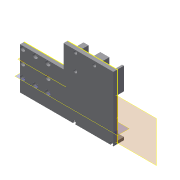
# Autodesk Inventor part: 10_MiniSPIM_Base_v1
Saved by Autodesk Inventor 2019 (Build 230136000, 136)
## iProperties
Created: 2019-10-10
Part Number: 10_MiniSPIM_Base_v1
Material: Generic
Document SubType Name: Modeling
Designer: diederichbenedict
Density: 1 g/cm^3
Appearance: Default
Author: diederichbenedict
Autodesk Inventor part; units mm, degrees
ref_plane "YZ Plane" through (0, 0, 0) normal (1, 0, 0) x (0, 1, 0)
ref_plane "XZ Plane" through (0, 0, 0) normal (0, 1, 0) x (-1, 0, 0)
ref_plane "XY Plane" through (0, 0, 0) normal (0, 0, 1) x (1, 0, 0)
ref_plane "Work Plane1" through (0, 0, 3) normal (0, 0, 1) x (1, 0, 0)
sketch "Sketch1" plane through (0, 0, 3) normal (0, 0, 1) x (1, 0, 0)
  line L0 (73, -36.65) -> (-73, -36.65) construction
  line L1 (73, 36.65) -> (73, -36.65) construction
  line L2 (-73, 36.65) -> (73, 36.65) construction
  line L3 (-73, -36.65) -> (-73, 36.65) construction
  line L4 (-66.8632, 12.8749) -> (-66.8632, 14.232) construction
  line L5 (-66.8632, 14.232) -> (-61.4969, 10.9795) construction
  line L6 (-61.4969, 10.9795) -> (-57.2382, 10.9795) construction
  line L7 (-57.2382, 10.9795) -> (-57.2382, 9.7003) construction
  line L8 (-57.2382, 9.7003) -> (-61.3643, 9.7003) construction
  line L9 (-61.3643, 9.7003) -> (-66.8632, 6.4478) construction
  line L10 (-66.8632, 6.4478) -> (-66.8632, 7.8674) construction
  line L11 (-66.8632, 7.8674) -> (-62.6279, 10.3477) construction
  line L12 (-62.6279, 10.3477) -> (-66.8632, 12.8749) construction
  spline S0 degree 2 poles (-57.9402, -12.888) (-57.519, -13.3482) (-57.0666, -14.5182) (-57.0666, -15.3995) knots 0 0 0 1 2 2 2 construction
  spline S1 degree 2 poles (-57.0666, -15.3995) (-57.0666, -16.4447) (-57.5034, -17.9111) (-57.8154, -18.5585) knots 0 0 0 1 2 2 2 construction
  line L13 (-57.8154, -18.5585) -> (-59.4221, -18.5585) construction
  line L14 (-59.4221, -18.5585) -> (-59.4221, -18.4649) construction
  spline S2 degree 2 poles (-59.4221, -18.4649) (-58.8294, -17.8331) (-58.1742, -16.2341) (-58.1742, -15.4931) knots 0 0 0 1 2 2 2 construction
  spline S3 degree 2 poles (-58.1742, -15.4931) (-58.1742, -14.4324) (-59.0555, -13.3482) (-59.7809, -13.3482) knots 0 0 0 1 2 2 2 construction
  spline S4 degree 2 poles (-59.7809, -13.3482) (-60.3581, -13.3482) (-61.0757, -13.9176) (-61.2551, -14.5338) knots 0 0 0 1 2 2 2 construction
  spline S5 degree 2 poles (-61.2551, -14.5338) (-61.3799, -14.9784) (-61.5515, -15.7193) (-61.6919, -16.2731) knots 0 0 0 1 2 2 2 construction
  spline S6 degree 2 poles (-61.6919, -16.2731) (-61.8245, -16.7723) (-62.2223, -17.5601) (-62.5421, -17.8643) knots 0 0 0 1 2 2 2 construction
  spline S7 degree 2 poles (-62.5421, -17.8643) (-62.8619, -18.1607) (-63.7199, -18.4883) (-64.2814, -18.4883) knots 0 0 0 1 2 2 2 construction
  spline S8 degree 2 poles (-64.2814, -18.4883) (-65.4514, -18.4883) (-67.0348, -16.6631) (-67.0348, -15.2514) knots 0 0 0 1 2 2 2 construction
  spline S9 degree 2 poles (-67.0348, -15.2514) (-67.0348, -14.4402) (-66.715, -13.005) (-66.4108, -12.3888) knots 0 0 0 1 2 2 2 construction
  line L15 (-66.4108, -12.3888) -> (-64.882, -12.3888) construction
  line L16 (-64.882, -12.3888) -> (-64.882, -12.4824) construction
  spline S10 degree 2 poles (-64.882, -12.4824) (-65.3032, -12.9426) (-65.9272, -14.3778) (-65.9272, -15.1656) knots 0 0 0 1 2 2 2 construction
  spline S11 degree 2 poles (-65.9272, -15.1656) (-65.9272, -16.0547) (-65.0926, -17.1545) (-64.414, -17.1545) knots 0 0 0 1 2 2 2 construction
  spline S12 degree 2 poles (-64.414, -17.1545) (-63.8057, -17.1545) (-63.0803, -16.5071) (-62.9165, -15.8987) knots 0 0 0 1 2 2 2 construction
  spline S13 degree 2 poles (-62.9165, -15.8987) (-62.8073, -15.4931) (-62.5265, -14.3154) (-62.4095, -13.9254) knots 0 0 0 1 2 2 2 construction
  spline S14 degree 2 poles (-62.4095, -13.9254) (-62.1053, -12.9348) (-60.8807, -12.0144) (-59.9837, -12.0144) knots 0 0 0 1 2 2 2 construction
  spline S15 degree 2 poles (-59.9837, -12.0144) (-59.4143, -12.0144) (-58.3224, -12.4746) (-57.9402, -12.888) knots 0 0 0 1 2 2 2 construction
  spline S16 degree 2 poles (-67.066, -7.0069) (-67.066, -6.0241) (-66.3796, -4.4486) (-65.7634, -3.9026) knots 0 0 0 1 2 2 2 construction
  spline S17 degree 2 poles (-65.7634, -3.9026) (-65.1238, -3.3566) (-63.2519, -2.7482) (-62.0507, -2.7482) knots 0 0 0 1 2 2 2 construction
  spline S18 degree 2 poles (-62.0507, -2.7482) (-60.8807, -2.7482) (-58.9854, -3.341) (-58.3458, -3.9026) knots 0 0 0 1 2 2 2 construction
  spline S19 degree 2 poles (-58.3458, -3.9026) (-57.675, -4.4954) (-57.0354, -6.0631) (-57.0354, -7.0069) knots 0 0 0 1 2 2 2 construction
  spline S20 degree 2 poles (-57.0354, -7.0069) (-57.0354, -7.9819) (-57.6984, -9.5419) (-58.3458, -10.1113) knots 0 0 0 1 2 2 2 construction
  spline S21 degree 2 poles (-58.3458, -10.1113) (-58.9854, -10.665) (-60.8651, -11.2578) (-62.0507, -11.2578) knots 0 0 0 1 2 2 2 construction
  spline S22 degree 2 poles (-62.0507, -11.2578) (-63.2597, -11.2578) (-65.1004, -10.6572) (-65.7634, -10.1035) knots 0 0 0 1 2 2 2 construction
  spline S23 degree 2 poles (-65.7634, -10.1035) (-66.403, -9.5419) (-67.066, -7.9741) (-67.066, -7.0069) knots 0 0 0 1 2 2 2 construction
  line L17 (-66.8632, 5.543) -> (-57.2382, 5.543) construction
  line L18 (-57.2382, 5.543) -> (-57.2382, 4.1078) construction
  line L19 (-57.2382, 4.1078) -> (-65.5372, -0.1509) construction
  line L20 (-65.5372, -0.1509) -> (-57.2382, -0.1509) construction
  line L21 (-57.2382, -0.1509) -> (-57.2382, -1.3442) construction
  line L22 (-57.2382, -1.3442) -> (-66.8632, -1.3442) construction
  line L23 (-66.8632, -1.3442) -> (-66.8632, 0.4731) construction
  line L24 (-66.8632, 0.4731) -> (-59.2427, 4.3496) construction
  line L25 (-59.2427, 4.3496) -> (-66.8632, 4.3496) construction
  line L26 (-66.8632, 4.3496) -> (-66.8632, 5.543) construction
  circle A0 centre (-154.415, -17.3382) radius 1.95 construction
  circle A1 centre (-129.415, 7.6618) radius 1.95 construction
  circle A2 centre (-129.415, 32.6618) radius 1.95 construction
  circle A3 centre (-179.415, -17.3382) radius 1.95 construction
  circle A4 centre (-179.415, 32.6618) radius 1.95 construction
  circle A5 centre (-129.415, -17.3382) radius 1.95 construction
  circle A6 centre (-179.415, 7.6618) radius 1.95 construction
  circle A7 centre (-154.415, 32.6618) radius 1.95 construction
  line L27 (-126.415, -22.3382) -> (-124.415, -20.3382) construction
  line L28 (-124.415, -20.3382) -> (-124.415, 35.6618) construction
  line L29 (-124.415, 35.6618) -> (-126.415, 37.6618) construction
  line L30 (-126.415, 37.6618) -> (-182.415, 37.6618) construction
  line L31 (-182.415, 37.6618) -> (-184.415, 35.6618) construction
  line L32 (-184.415, 35.6618) -> (-184.415, -20.3382) construction
  line L33 (-184.415, -20.3382) -> (-182.415, -22.3382) construction
  line L34 (-182.415, -22.3382) -> (-126.415, -22.3382) construction
  circle A8 centre (-93.2, 28.85) radius 2.1512 construction
  arc A9 (-95.5, 82.55) -> (-98.5, 79.55) centre (-95.5, 79.55) ccw construction
  line L35 (-98.5, 18.65) -> (-98.5, 79.55) construction
  arc A10 (-98.5, 18.65) -> (-95.5, 15.65) centre (-95.5, 18.65) ccw construction
  line L36 (39.6, 15.65) -> (-95.5, 15.65) construction
  arc A11 (39.6, 15.65) -> (42.6, 18.65) centre (39.6, 18.65) ccw construction
  line L37 (42.6, 79.55) -> (42.6, 18.65) construction
  arc A12 (42.6, 79.55) -> (39.6, 82.55) centre (39.6, 79.55) ccw construction
  line L38 (-95.5, 82.55) -> (39.6, 82.55) construction
  line L39 (-184.415, -44.9655) -> (0, -44.9655)
  line L40 (0, -44.9655) -> (0, 82.55)
  line L41 (0, 82.55) -> (-184.415, 82.55)
  line L42 (-184.415, 82.55) -> (-184.415, -44.9655)
  circle A13 centre (-179.415, 32.6618) radius 2.95
  circle A14 centre (-154.415, 32.6618) radius 2.95
  circle A15 centre (-129.415, 32.6618) radius 2.95
  circle A16 centre (-129.415, 7.6618) radius 2.95
  circle A17 centre (-129.415, -17.3382) radius 2.95
  circle A18 centre (-154.415, -17.3382) radius 2.95
  circle A19 centre (-179.415, -17.3382) radius 2.95
  circle A20 centre (-179.415, 7.6618) radius 2.95
  line L43 (-184.415, 82.55) -> (-98.5, 82.55)
  line L44 (-98.5, 82.55) -> (-98.5, 37.6618)
  line L45 (-98.5, 37.6618) -> (-184.415, 37.6618)
  line L46 (-184.415, 37.6618) -> (-184.415, 82.55)
  point P0 (0, 0)
  dimension "d0" = 1
  dimension "d1" = 1
  dimension "d2" = 1
  dimension "d3" = 1
  dimension "d4" = 1
  dimension "d5" = 1
  dimension "d6" = 1
  dimension "d7" = 1
  constraints: 16 end point, 8 centre point, 4 parallel, 2 horizontal, 2 perpendicular, 2 point on line
  measures "d0" radial gap between concentric circles of A4 A13
  measures "d1" radial gap between concentric circles of A7 A14
  measures "d2" radial gap between concentric circles of A2 A15
  measures "d3" radial gap between concentric circles of A1 A16
  measures "d4" radial gap between concentric circles of A5 A17
  measures "d5" radial gap between concentric circles of A0 A18
  measures "d6" radial gap between concentric circles of A3 A19
  measures "d7" radial gap between concentric circles of A6 A20
ref_plane "Work Plane2" through (-73, -36.65, 0) normal (0, 0, 1) x (1, 0, 0)
extrude "Extrusion1" add sketch "Sketch1" along normal blind 5 and the other way blind 3 contours L42 L45 L44 L41 L40 L39
sketch "Sketch2" plane through (0, 0, 0) normal (0, 0, -1) x (1, 0, 0)
  line L0 (-184.415, -37.6618) -> (-98.5, -37.6618) projected
  line L1 (-184.415, 44.9655) -> (-184.415, -37.6618) projected
  line L2 (0, 44.9655) -> (-184.415, 44.9655) projected
  line L3 (0, -82.55) -> (0, 44.9655) projected
  line L4 (-98.5, -82.55) -> (0, -82.55) projected
  line L5 (-98.5, -37.6618) -> (-98.5, -82.55) projected
  circle A0 centre (-179.415, -7.6618) radius 2.95 projected
  circle A1 centre (-179.415, 17.3382) radius 2.95 projected
  circle A2 centre (-154.415, 17.3382) radius 2.95 projected
  circle A3 centre (-129.415, 17.3382) radius 2.95 projected
  circle A4 centre (-129.415, -7.6618) radius 2.95 projected
  circle A5 centre (-129.415, -32.6618) radius 2.95 projected
  circle A6 centre (-154.415, -32.6618) radius 2.95 projected
  circle A7 centre (-179.415, -32.6618) radius 2.95 projected
  point P0 (0, 0)
sketch "Sketch3" plane through (0, 0, 8) normal (0, 0, 1) x (1, 0, 0)
  line L0 (-98.5, 82.55) -> (-98.5, 37.6618) projected
  line L1 (-98.5, 37.6618) -> (-184.415, 37.6618) projected
  line L2 (-184.415, 37.6618) -> (-184.415, -44.9655) projected
  line L3 (-184.415, -44.9655) -> (0, -44.9655) projected
  line L4 (0, -44.9655) -> (0, 82.55) projected
  line L5 (0, 82.55) -> (-98.5, 82.55) projected
  circle A0 centre (-179.415, 32.6618) radius 2.95 projected
  circle A1 centre (-154.415, 32.6618) radius 2.95 projected
  circle A2 centre (-129.415, 32.6618) radius 2.95 projected
  circle A3 centre (-129.415, 7.6618) radius 2.95 projected
  circle A4 centre (-129.415, -17.3382) radius 2.95 projected
  circle A5 centre (-154.415, -17.3382) radius 2.95 projected
  circle A6 centre (-179.415, -17.3382) radius 2.95 projected
  circle A7 centre (-179.415, 7.6618) radius 2.95 projected
  point P0 (0, 0)
hole "Hole1" at (-179.415, 32.6618, 8) at (-154.415, 32.6618, 8) at (-129.415, 32.6618, 8) at (-129.415, 7.6618, 8) at (-129.415, -17.3382, 8) at (-154.415, -17.3382, 8) at (-179.415, -17.3382, 8) at (-179.415, 7.6618, 8) direction (0, 0, -1) diameter 5.3 depth 10 tip angle 118 counterbore diameter 10 counterbore depth 5
sketch "Sketch4" plane through (0, 0, 0) normal (0, 0, -1) x (-1, 0, 0)
  line L0 (-75, -38.65) -> (75, -38.65) projected
  line L1 (75, 38.65) -> (-75, 38.65) projected
  line L2 (0, -44.9655) -> (184.415, -44.9655) projected
  line L3 (0, -44.9655) -> (75, -44.9655)
  line L4 (75, -44.9655) -> (75, -39.3793)
  line L5 (75, -39.3793) -> (0, -39.3793)
  line L6 (0, -39.3793) -> (0, -44.9655)
  line L7 (98.5, 82.55) -> (0, 82.55) projected
  line L8 (0, 82.55) -> (3.6448, 82.55)
  line L9 (3.6448, 82.55) -> (3.6448, 38.65)
  line L10 (3.6448, 38.65) -> (0, 38.65)
  line L11 (0, 38.65) -> (0, 82.55)
  line L12 (33.963, 38.65) -> (28.963, 38.65)
  line L13 (28.963, 38.65) -> (28.963, 82.55)
  line L14 (28.963, 82.55) -> (33.963, 82.55)
  line L15 (33.963, 82.55) -> (33.963, 38.65)
  line L16 (70, 38.65) -> (75, 38.65)
  line L17 (75, 38.65) -> (75, 82.55)
  line L18 (75, 82.55) -> (70, 82.55)
  line L19 (70, 82.55) -> (70, 38.65)
  line L20 (75, -44.9655) -> (80, -44.9655)
  line L21 (80, -44.9655) -> (80, -8.9655)
  line L22 (80, -8.9655) -> (75, -8.9655)
  line L23 (75, -8.9655) -> (75, -44.9655)
  line L24 (75, 82.55) -> (80, 82.55)
  line L25 (80, 82.55) -> (80, 32.55)
  line L26 (80, 32.55) -> (75, 32.55)
  line L27 (75, 32.55) -> (75, 82.55)
  line L28 (0, 38.65) -> (75, 38.65)
  line L29 (75, 38.65) -> (75, 39.65)
  line L30 (75, 39.65) -> (0, 39.65)
  line L31 (0, 39.65) -> (0, 38.65)
  line L32 (75, -8.9655) -> (107, -8.9655)
  line L33 (107, -8.9655) -> (107, -3.9655)
  line L34 (107, -3.9655) -> (75, -3.9655)
  line L35 (75, -3.9655) -> (75, -8.9655)
  line L36 (33.963, 82.55) -> (46.7902, 82.55)
  line L37 (46.7902, 82.55) -> (46.7902, 67.4779)
  line L38 (46.7902, 67.4779) -> (33.963, 67.4779)
  line L39 (33.963, 67.4779) -> (33.963, 82.55)
  point P0 (0, 0)
  point P1 (70, 39.65)
  point P2 (33.963, 39.65)
  point P3 (28.963, 39.65)
  point P4 (3.6448, 39.65)
  dimension "d19" = 5
  dimension "d20" = 36
  dimension "d21" = 50
  dimension "d22" = 5
  dimension "d23" = 5
  dimension "d24" = 1
  dimension "d41" = 32
  dimension "d42" = 5
  constraints: 72 end point, 18 parallel, 16 point on line, 9 horizontal, 9 perpendicular, 1 coincident
  measures "d19" distance of L22.end L21.end
  measures "d20" distance of L21.end L20.end
  measures "d21" distance of L24.end L25.end
  measures "d22" distance between parallel lines of L13 L15
  measures "d23" distance between parallel lines of L19 L17
  measures "d24" distance of L29.end L28.end
  measures "d41" distance of L34.end L33.end
  measures "d42" distance of L33.end L32.end
ref_plane "Work Plane3" through (-73, -36.65, -13.1) normal (0, 0, -1) x (0, 1, 0)
extrude "Extrusion2" add sketch "Sketch4" along normal up to surface (13.1 mm away) contours L1 L19 L30 L17 | L17 L7 L25 L26 L27 | L1 L15 L30 L19 | L30 L19 L7 L17 | L1 L13 L30 L15 | L1 L9 L30 L13 | L30 L13 L7 L15 | L1 L11 L30 L9 | L15 L7 L37 L38 | L30 L11 L7 L9 | L6 L5 L4 L2 | L4 L23 L22 L21 L2 | L22 L35 L34 L33 L32
ref_plane "Work Plane4" through (-184.415, -21.1655, 8) normal (0, -1, 0) x (1, 0, 0)
sketch "Sketch5" plane through (-184.415, -21.1655, 8) normal (0, -1, 0) x (1, 0, 0)
  line L0 (106.215, -7.26) -> (106.215, -19.94) projected
  arc A0 (109.315, -13.6) -> (107.415, -7.26) centre (94.5273, -14.5769) ccw
  arc A1 (107.415, -19.94) -> (109.315, -13.6) centre (94.5273, -12.6231) ccw
  line L1 (107.415, -7.26) -> (106.215, -7.26)
  line L2 (107.415, -19.94) -> (106.215, -19.94)
  arc A2 (109.6156, -13.6) -> (107.5884, -6.96) centre (94.5273, -14.5769) ccw
  line L3 (107.5884, -6.96) -> (105.915, -6.96)
  line L4 (105.915, -6.96) -> (105.915, -20.24)
  line L5 (105.915, -20.24) -> (107.5884, -20.24)
  arc A3 (107.5884, -20.24) -> (109.6156, -13.6) centre (94.5273, -12.6231) ccw
  line L6 (105.915, -19.2866) -> (104.415, -19.2866)
  line L7 (104.415, -8) -> (104.415, -21.1) projected
  line L8 (104.415, -13.6) -> (105.915, -13.6)
  line L9 (108.0996, -19.2866) -> (109.415, -19.2866)
  line L10 (109.415, -8) -> (109.415, -21.1) projected
  line L11 (105.915, -13.6) -> (109.6156, -13.6)
  line L12 (104.415, -8) -> (105.915, -8)
  line L13 (108.1418, -8) -> (109.415, -8)
  line L14 (109.415, -8) -> (109.415, -11.9371)
  line L15 (109.415, -11.9371) -> (109.415, -13.6)
  arc A4 (105.915, -6.96) -> (105.915, -20.24) centre (128.582, -13.6) ccw
  line L16 (104.9624, -13.6) -> (105.915, -13.6)
  line L17 (106.215, -7.26) -> (105.915, -7.26)
  line L18 (106.215, -19.94) -> (105.915, -19.94)
  point P0 (184.415, -8)
  dimension "d28" = 0.3
  constraints: 32 end point, 14 point on circle, 11 point on line, 5 centre point, 4 horizontal, 2 collinear, 2 parallel, 2 perpendicular, 1 coincident, 1 midpoint, 11 other
  measures "d28" radial gap between concentric circles of A1 A3
revolve "Revolution1" cut sketch "Sketch5" angle 360 about axis through (-80, -21.1655, -5.6) along (1, 0, 0) contours L1 A0 L11 L0 | L17 L4 L3 A2 L10 L11 A0 L1 | L0 L11 L4 L17 | L8 A4 L12 L4 | L8 L7 L12 A4 | L10 A2 L11 | A2 L13 L10
sketch "Sketch6" plane through (0, -44.9655, -13.1) normal (0, 0, -1) x (-1, 0, 0)
  line L0 (78.5, 17.16) -> (78.5, 30.44) projected
  line L1 (76.8265, 17.16) -> (78.5, 17.16) projected
  line L2 (76.8265, 30.44) -> (78.5, 30.44) projected
  arc A0 (77, 30.1555) -> (75.1, 23.8155) centre (89.8876, 22.8386) ccw
  arc A1 (75.1, 23.8155) -> (77, 17.4755) centre (89.8876, 24.7925) ccw
  line L3 (76.2622, 30.8555) -> (79.2, 30.8555)
  line L4 (79.2, 30.8555) -> (79.2, 16.46)
  line L5 (79.2, 16.46) -> (76.2622, 16.46)
  line L6 (76.2622, 16.46) -> (76.2622, 30.8555)
  line L7 (76.2622, 30.8555) -> (79.2, 16.46) construction
  line L8 (79.2, 30.8555) -> (76.2622, 16.46) construction
  arc A2 (76.2622, 30.8555) -> (76.2622, 16.46) centre (91.2579, 23.6578) ccw
  arc A3 (78.5, 16.46) -> (78.5, 30.8555) centre (55.9892, 23.6578) ccw
  point P0 (0, 44.9655)
  point P1 (77.7311, 23.6578)
  dimension "d30" = 0.7
  dimension "d31" = 0.7
  dimension "d32" = 0.7
  constraints: 12 end point, 8 point on circle, 4 centre point, 2 midpoint, 2 parallel, 2 point on line, 1 horizontal, 1 perpendicular, 7 other
  measures "d30" distance between parallel lines of L1 L5
  measures "d31" distance from line of L3 A0.start
  measures "d32" distance between parallel lines of L4 L0
extrude "Extrusion3" cut sketch "Sketch6" against normal blind 7
ref_plane "Work Plane5" through (-184.415, 10.1618, 0) normal (0, 1, 0) x (1, 0, 0)
sketch "Sketch8" plane through (0, 0, 0) normal (0, 0, -1) x (-1, 0, 0)
  point P0 (0, 0)
ref_plane "Work Plane6" through (-92.97, -44.9655, -13.1) normal (-1, 0, 0) x (0, 0, 1)
sketch "Sketch9" plane through (-92.97, -44.9655, -13.1) normal (-1, 0, 0) x (0, 0, 1)
  line L0 (1.5, 45.9155) -> (1.5, 30.5155) construction
  line L1 (-1.25, 45.9155) -> (16.25, 45.9155) construction
  line L2 (-1.25, 50.6155) -> (-1.25, 45.9155) construction
  arc A0 (7, 53.5251) -> (-1.25, 50.6155) centre (7, 40.3737) ccw construction
  line L3 (1.5, 30.5155) -> (13.5, 30.5155) construction
  line L4 (13.5, 45.9155) -> (13.5, 30.5155) construction
  arc A1 (16.25, 50.6155) -> (8, 53.5251) centre (8, 40.3737) ccw construction
  line L5 (13.1, 41) -> (0, 41) projected
  line L6 (7.5, 23.7837) -> (1.5, 23.7837)
  line L7 (1.5, 23.7837) -> (1.5, 41)
  line L8 (1.5, 41) -> (7.5, 41)
  line L9 (7.5, 41) -> (7.5, 23.7837)
  line L10 (7.5, 41) -> (-4.503, 41)
  line L11 (-4.503, 41) -> (-4.503, 60.9686)
  line L12 (-4.503, 60.9686) -> (7.5, 60.9686)
  line L13 (7.5, 60.9686) -> (7.5, 41)
  point P0 (13.1, 44.9655)
  constraints: 22 end point, 4 parallel, 4 point on circle, 3 vertical, 2 centre point, 2 horizontal, 2 perpendicular, 2 point on line, 11 other
revolve "Revolution2" cut sketch "Sketch9" angle 360 about axis through (-92.97, -3.9655, -5.6) along (0, -1, 0)
sketch "Sketch10" plane through (-80, 32.55, 0) normal (-1, 0, 0) x (0, 0, 1)
  line L0 (-1.3574, -6.5284) -> (-8.4284, 0.5426) projected
  line L1 (0, -77.5155) -> (0, 5.1118) projected
  line L2 (0, -7.8858) -> (-12.9976, 5.1118)
  line L3 (-12.9976, 5.1118) -> (0, 5.1118)
  line L4 (0, 5.1118) -> (0, -7.8858)
  point P0 (0, -32.55)
  constraints: 6 end point, 1 collinear, 1 perpendicular, 1 point on line
extrude "Extrusion5" add sketch "Sketch10" along normal up to surface (18.5 mm away)
sketch "Sketch11" plane through (0, 0, 8) normal (0, 0, 1) x (1, 0, 0)
  circle A0 centre (-154.415, -17.3382) radius 5 projected
  circle A1 centre (-129.415, 7.6618) radius 5 projected
  circle A2 centre (-129.415, -17.3382) radius 5 projected
  arc A3 (-184.415, 32.6618) -> (-179.415, 37.6618) centre (-179.415, 32.6618) ccw projected
  line L0 (-184.415, 32.6618) -> (-184.415, 7.6618) projected
  circle A4 centre (-179.415, 7.6618) radius 5 projected
  line L1 (-184.415, 7.6618) -> (-184.415, -17.3382) projected
  circle A5 centre (-179.415, -17.3382) radius 5 projected
  line L2 (-184.415, -17.3382) -> (-184.415, -44.9655) projected
  line L3 (-184.415, -44.9655) -> (0, -44.9655) projected
  line L4 (0, -44.9655) -> (0, 82.55) projected
  line L5 (0, 82.55) -> (-98.5, 82.55) projected
  line L6 (-98.5, 82.55) -> (-98.5, 37.6618) projected
  line L7 (-98.5, 37.6618) -> (-129.415, 37.6618) projected
  circle A6 centre (-129.415, 32.6618) radius 5 projected
  line L8 (-129.415, 37.6618) -> (-154.415, 37.6618) projected
  circle A7 centre (-154.415, 32.6618) radius 5 projected
  line L9 (-154.415, 37.6618) -> (-179.415, 37.6618) projected
  line L10 (-28.963, 82.55) -> (-46.7902, 82.55) projected
  line L11 (-28.963, 39.65) -> (-28.963, 82.55) projected
  line L12 (-3.6448, 39.65) -> (-28.963, 39.65) projected
  line L13 (-3.6448, 82.55) -> (-3.6448, 39.65) projected
  line L14 (0, 82.55) -> (-3.6448, 82.55) projected
  line L15 (0, 38.65) -> (0, 82.55) projected
  line L16 (-75, 38.65) -> (0, 38.65) projected
  line L17 (-75, 32.55) -> (-75, 38.65) projected
  line L18 (-80, 32.55) -> (-75, 32.55) projected
  line L19 (-80, 82.55) -> (-80, 32.55) projected
  line L20 (-70, 82.55) -> (-80, 82.55) projected
  line L21 (-70, 39.65) -> (-70, 82.55) projected
  line L22 (-33.963, 39.65) -> (-70, 39.65) projected
  line L23 (-33.963, 67.4779) -> (-33.963, 39.65) projected
  arc A8 (-75, -17.7921) -> (-76.2622, -14.11) centre (-91.2579, -21.3078) ccw projected
  line L24 (-76.2622, -14.11) -> (-79.2, -14.11) projected
  line L25 (-79.2, -14.11) -> (-79.2, -16.8577) projected
  arc A9 (-79.2, -16.8577) -> (-79.2, -25.7578) centre (-55.9892, -21.3078) ccw projected
  line L26 (-79.2, -25.7578) -> (-79.2, -28.5055) projected
  line L27 (-79.2, -28.5055) -> (-76.2622, -28.5055) projected
  arc A10 (-76.2622, -28.5055) -> (-75, -24.8235) centre (-91.2579, -21.3078) ccw projected
  line L28 (-75, -39.3793) -> (-75, -24.8235) projected
  line L29 (0, -39.3793) -> (-75, -39.3793) projected
  line L30 (0, -44.9655) -> (0, -39.3793) projected
  line L31 (-80, -44.9655) -> (0, -44.9655) projected
  line L32 (-80, -8.9655) -> (-80, -44.9655) projected
  line L33 (-107, -8.9655) -> (-80, -8.9655) projected
  line L34 (-107, -3.9655) -> (-107, -8.9655) projected
  line L35 (-75, -3.9655) -> (-107, -3.9655) projected
  line L36 (-75, -17.7921) -> (-75, -3.9655) projected
  line L37 (-46.7902, 67.4779) -> (-33.963, 67.4779) projected
  line L38 (-46.7902, 82.55) -> (-46.7902, 67.4779) projected
  point P0 (0, 0)
  point P1 (-75, 78.2799)
  point P2 (-75, 46.097)
  point P3 (-77.7311, -42.1724)
  point P4 (-3.6448, -42.1724)
  point P5 (-37.5, 75.014)
  constraints: 2 horizontal alignment, 2 vertical alignment
hole "Hole2" at (-75, 78.2799, 8) at (-75, 46.097, 8) at (-77.7311, -42.1724, 8) at (-3.6448, -42.1724, 8) at (-37.5, 75.014, 8) direction (0, 0, -1) diameter 3.3 end through all counterbore diameter 6.8 counterbore depth 5
sketch "Sketch12" plane through (0, 0, 0) normal (0, 0, -1) x (-1, 0, 0)
  line L0 (80, 24.6642) -> (80, 32.55) projected
  line L1 (80, 32.55) -> (75, 32.55) projected
  line L2 (75, 32.55) -> (75, 38.65) projected
  line L3 (75, 38.65) -> (0, 38.65) projected
  line L4 (0, 38.65) -> (0, -39.3793) projected
  line L5 (0, -39.3793) -> (75, -39.3793) projected
  line L6 (75, -39.3793) -> (75, -21.1655) projected
  line L7 (75, -21.1655) -> (75, -3.9655) projected
  line L8 (75, -3.9655) -> (82.3534, -3.9655) projected
  line L9 (82.3534, -3.9655) -> (82.3534, 16.003) projected
  line L10 (82.3534, 16.003) -> (103.5866, 16.003) projected
  line L11 (103.5866, 16.003) -> (103.5866, -3.9655) projected
  line L12 (103.5866, -3.9655) -> (107, -3.9655) projected
  line L13 (107, -3.9655) -> (107, -8.9655) projected
  line L14 (107, -8.9655) -> (95.1241, -8.9655) projected
  line L15 (95.1241, -8.9655) -> (95.1241, -21.1818) projected
  line L16 (95.1241, -21.1818) -> (90.8159, -21.1818) projected
  line L17 (90.8159, -21.1818) -> (90.8159, -8.9655) projected
  line L18 (90.8159, -8.9655) -> (80, -8.9655) projected
  line L19 (80, -8.9655) -> (80, -21.1655) projected
  line L20 (80, -21.1655) -> (80, -44.9655) projected
  line L21 (80, -44.9655) -> (184.415, -44.9655) projected
  line L22 (184.415, -44.9655) -> (184.415, 37.6618) projected
  line L23 (184.415, 37.6618) -> (98.5, 37.6618) projected
  line L24 (98.5, 37.6618) -> (98.5, 24.6642) projected
  line L25 (98.5, 24.6642) -> (80, 24.6642) projected
  circle A0 centre (179.415, 7.6618) radius 2.95 projected
  circle A1 centre (179.415, -17.3382) radius 2.95 projected
  circle A2 centre (154.415, -17.3382) radius 2.95 projected
  circle A3 centre (129.415, -17.3382) radius 2.95 projected
  circle A4 centre (129.415, 7.6618) radius 2.95 projected
  circle A5 centre (129.415, 32.6618) radius 2.95 projected
  circle A6 centre (154.415, 32.6618) radius 2.95 projected
  circle A7 centre (179.415, 32.6618) radius 2.95 projected
  line L26 (126.415, -22.3382) -> (124.415, -20.3382) projected
  line L27 (126.415, -22.3382) -> (182.415, -22.3382) projected
  line L28 (184.415, -20.3382) -> (182.415, -22.3382) projected
  line L29 (184.415, -20.3382) -> (184.415, 35.6618) projected
  line L30 (182.415, 37.6618) -> (184.415, 35.6618) projected
  line L31 (182.415, 37.6618) -> (126.415, 37.6618) projected
  line L32 (124.415, 35.6618) -> (126.415, 37.6618) projected
  line L33 (124.415, 35.6618) -> (124.415, -20.3382) projected
  circle A8 centre (129.415, 7.6618) radius 1.3 projected
  circle A9 centre (179.415, 7.6618) radius 1.3 projected
  circle A10 centre (154.415, 7.6618) radius 7.5 projected
  line L34 (107, -8.9655) -> (80, -8.9655) projected
  line L35 (184.415, -44.9655) -> (79.6698, -44.9655) projected
  line L36 (80, -8.9655) -> (124.415, -8.9655)
  line L37 (124.415, -8.9655) -> (124.415, -44.9655)
  line L38 (124.415, -44.9655) -> (80, -44.9655)
  line L39 (80, -44.9655) -> (80, -8.9655)
  line L40 (184.415, -44.9655) -> (124.415, -44.9655)
  line L41 (124.415, -44.9655) -> (124.415, -22.3382)
  line L42 (124.415, -22.3382) -> (184.415, -22.3382)
  line L43 (184.415, -22.3382) -> (184.415, -44.9655)
  line L44 (90.8159, -21.1818) -> (95.1241, -21.1818)
  line L45 (95.1241, -21.1818) -> (95.1241, -8.9655)
  line L46 (95.1241, -8.9655) -> (90.8159, -8.9655)
  line L47 (90.8159, -8.9655) -> (90.8159, -21.1818)
  point P0 (0, 0)
  constraints: 24 end point, 6 parallel, 3 horizontal, 3 perpendicular, 2 point on line
extrude "Extrusion6" cut sketch "Sketch12" against normal blind 4 contours L33 L37 L21 L20 L19 L18 L17 L16 L15 L14 L36 | L22 L21 L37 L42 L27 | L15 L16 L17 L34
body "Solid1"
